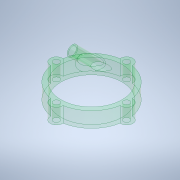
# Autodesk Inventor part: Central
Saved by Autodesk Inventor 2020 (Build 240168000, 168)
## iProperties
Created: 2020-10-28
Part Number: Central
Material: Generic
Document SubType Name: Modeling
Designer: aaron
Density: 1 g/cm^3
Appearance: Clear - Green 1
Author: aaron
Autodesk Inventor part; units mm, degrees
ref_plane "YZ Plane" through (0, 0, 0) normal (1, 0, 0) x (0, 1, 0)
ref_plane "XZ Plane" through (0, 0, 0) normal (0, 1, 0) x (-1, 0, 0)
ref_plane "XY Plane" through (0, 0, 0) normal (0, 0, 1) x (1, 0, 0)
sketch "Sketch1" plane through (0, 0, 0) normal (0, 1, 0) x (-1, 0, 0)
  circle A0 centre (0, 0) radius 12.5 construction
  line L0 (12.5, 0) -> (-12.5, 0) construction
  line L1 (0, -12.5) -> (0, 12.5) construction
  circle A1 centre (-11.5, 0) radius 1
  circle A2 centre (0, -11.5) radius 1
  circle A3 centre (11.5, 0) radius 1
  circle A4 centre (0, 11.5) radius 1
  circle A5 centre (0, 0) radius 10
  arc A6 (-1.9924, -11.3261) -> (1.9924, -11.3261) centre (0, -11.5) ccw
  arc A7 (-11.3261, 1.9924) -> (-11.3261, -1.9924) centre (-11.5, 0) ccw
  arc A8 (1.9924, 11.3261) -> (-1.9924, 11.3261) centre (0, 11.5) ccw
  arc A9 (11.3261, -1.9924) -> (11.3261, 1.9924) centre (11.5, 0) ccw
  arc A10 (0.9991, -11.4565) -> (11.3261, -1.9924) centre (0, 0) ccw construction
  arc A11 (1.9924, -11.3261) -> (11.3261, -1.9924) centre (0, 0) ccw
  arc A12 (11.3261, 1.9924) -> (1.9924, 11.3261) centre (0, 0) ccw construction
  arc A13 (11.3261, 1.9924) -> (1.9924, 11.3261) centre (0, 0) ccw
  arc A14 (-1.9924, 11.3261) -> (-11.3261, 1.9924) centre (0, 0) ccw construction
  arc A15 (-1.9924, 11.3261) -> (-11.3261, 1.9924) centre (0, 0) ccw
  arc A16 (-11.3261, -1.9924) -> (-1.9924, -11.3261) centre (0, 0) ccw construction
  arc A17 (-11.3261, -1.9924) -> (-1.9924, -11.3261) centre (0, 0) ccw
  line L2 (0, -10) -> (-12.5, -10) construction
  dimension "d2" = 2
  dimension "d3" = 20
  dimension "d0" = 25
  dimension "d5" = 2
  dimension "d6" = 11.5
  dimension "d7" = 11.5
  dimension "d8" = 11.5
  dimension "d9" = 11.5
  constraints: 28 point on circle, 13 centre point, 8 coincident, 6 end point, 5 point on line, 3 equal radius, 3 horizontal, 2 horizontal alignment, 2 vertical alignment, 1 perpendicular, 14 other
  measures "d0" diameter of A0
  measures "d5" radius of A9
  measures "d6" radius of A16
  measures "d7" radius of A14
  measures "d8" radius of A12
  measures "d9" radius of A10
extrude "Extrusion1" add sketch "Sketch1" along normal blind 5
ref_plane "Work Plane1" through (-11.5, 0, 0) normal (-1, 0, 0) x (0, -1, 0)
sketch "Sketch2" plane through (-11.5, 0, 0) normal (-1, 0, 0) x (0, -1, 0)
  line L0 (0, 10) -> (0, -10) projected
  line L1 (0, -10) -> (-5, -10) construction
  line L2 (-5, -10) -> (0, -10) construction
  line L3 (-2.5, -10) -> (-2.5, -1.9924) construction
  line L4 (0, -1.9924) -> (-5, -1.9924) construction
  circle A0 centre (-2.5, -8.25) radius 1.75
  point P0 (0, 0)
  dimension "d12" = 5
  dimension "d13" = 3.5
  constraints: 4 end point, 2 midpoint, 1 centre point, 1 horizontal, 1 point on line, 1 tangent
  measures "d12" distance of L0.end L1.end
  measures "d13" diameter of A0
extrude "Extrusion2" add sketch "Sketch2" against normal up to surface round surface about axis through (0, 0, 0) along (0, 1, 0) radius 10 far side no
sketch "Sketch4" plane through (-11.5, 2.5, -8.25) normal (-1, 0, 0) x (0, 0, 1)
  circle A0 centre (0, 0) radius 1.75 projected
  circle A1 centre (0, 0) radius 1.3
  point P0 (8.25, -2.5)
  dimension "d16" = 2.6
  constraints: 1 centre point, 1 coincident
  measures "d16" diameter of A1
extrude "Extrusion3" cut sketch "Sketch4" against normal up to surface contours A1 round surface about axis through (0, 0, 0) along (0, 1, 0) radius 10 far side no
sketch "Sketch5" plane through (-11.5, 2.5, -8.25) normal (-1, 0, 0) x (0, 0, 1)
  circle A0 centre (0, 0) radius 1.3 projected
  circle A1 centre (0, 0) radius 1.75 projected
  point P0 (8.25, -2.5)
extrude "Extrusion4" add sketch "Sketch5" along normal blind 3
fillet "Fillet1" radius 1 1 edges at (-7.613, 4.2106, -8.6193)
body "Solid1"
